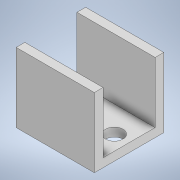
# Autodesk Inventor part: halfinchCChannel
Saved by Autodesk Inventor 2021 (Build 250183000, 183)
## iProperties
Created: 2021-12-02
Part Number: halfinchCChannel
Material: Generic
Document SubType Name: Modeling
Designer: Unit-005
Density: 1 g/cm^3
Appearance: Default
Author: Unit-005
Autodesk Inventor part; units mm, degrees
ref_plane "YZ Plane" through (0, 0, 0) normal (1, 0, 0) x (0, 1, 0)
ref_plane "XZ Plane" through (0, 0, 0) normal (0, 1, 0) x (-1, 0, 0)
ref_plane "XY Plane" through (0, 0, 0) normal (0, 0, 1) x (1, 0, 0)
sketch "Sketch2" plane through (0, 0, 0) normal (1, 0, 0) x (0, 1, 0)
  line L0 (-6.35, 6.35) -> (6.35, 6.35)
  line L1 (6.35, 6.35) -> (6.35, -6.35)
  line L2 (6.35, -6.35) -> (-6.35, -6.35)
  line L3 (-6.35, -6.35) -> (-6.35, 6.35)
  line L4 (-6.35, 6.35) -> (6.35, -6.35) construction
  line L5 (6.35, 6.35) -> (-6.35, -6.35) construction
  line L6 (-4.7625, 4.7625) -> (4.7625, 4.7625)
  line L7 (4.7625, 4.7625) -> (4.7625, -4.7625)
  line L8 (4.7625, -4.7625) -> (-4.7625, -4.7625)
  line L9 (-4.7625, -4.7625) -> (-4.7625, 4.7625)
  line L10 (-4.7625, 4.7625) -> (4.7625, -4.7625) construction
  line L11 (4.7625, 4.7625) -> (-4.7625, -4.7625) construction
  line L12 (4.7625, 4.7625) -> (6.35, 4.7625)
  line L13 (4.7625, -4.7625) -> (6.35, -4.7625)
  point P0 (0, 0)
  dimension "d0" = 12.7
  dimension "d1" = 12.7
  dimension "d2" = 9.525
  dimension "d3" = 9.525
  constraints: 28 end point, 5 parallel, 4 midpoint, 3 horizontal, 2 perpendicular, 2 point on line
  measures "d0" distance of L1.end L2.end
  measures "d1" distance of L0.end L1.end
  measures "d2" distance of L7.end L8.end
  measures "d3" distance of L6.end L7.end
extrude "Extrusion1" add sketch "Sketch2" along normal mid plane 14.2875 contours L0 L1 L12 L6 L9 L8 L13 L2 L3
sketch "Sketch3" plane through (-7.1437, -4.7625, 4.7625) normal (0, 1, 0) x (1, 0, 0)
  line L0 (0, 0) -> (14.2875, 0) projected
  line L1 (14.2875, 9.525) -> (14.2875, 0) projected
  line L2 (0, 9.525) -> (14.2875, 9.525) projected
  line L3 (0, 0) -> (0, 9.525) projected
  line L4 (-2.8575, 4.7625) -> (17.145, 4.7625) projected
  line L5 (7.1437, 13.6525) -> (7.1437, -4.1275) projected
  circle A0 centre (2.6988, 4.7625) radius 1.5875
  point P0 (7.1437, 4.7625)
  dimension "d6" = 3.175
  dimension "d7" = 4.445
  constraints: 1 centre point, 1 point on line
  measures "d6" diameter of A0
  measures "d7" distance from line of L5 A0.centre
extrude "Extrusion2" cut sketch "Sketch3" against normal through all contours A0 L4 | L4 A0
mirror "Mirror1" about plane through (0, 0, 0) normal (1, 0, 0) of "Extrusion2"
body "Solid1"
